Autodesk Fusion 360 part; units mm, degrees
note: some values were not read from the file. Chosen so that the rebuilt part matches the saved one: which face or edge a step refers to; which pieces of a blend or face edit are solid.
(part 2 of 2)
extrude "Extrusion30" add sketch "Skizze30" along normal blind 1 contours L54 L59 L60 L61 L62 L63 bodies 1
sketch "Skizze31" plane through (0, 1, 0) normal (0, 1, 0) x (-1, 0, 0)
  line L0 (-3.5, 38.5) -> (-3.5, 36.5)
  line L1 (-3.5, 36.5) -> (-5.5, 36.5)
  line L2 (-5.5, 36.5) -> (-5.5, 34)
  line L3 (-5.5, 34) -> (-6, 34)
  line L4 (-6, 34) -> (-6, 39)
  line L5 (-6, 39) -> (-1, 39)
  line L6 (-1, 39) -> (-1, 38.5)
  line L7 (-1, 38.5) -> (-3.5, 38.5)
  line L8 (10.5, 34) -> (10.5, 38.5)
  line L9 (10.5, 38.5) -> (6, 38.5)
  line L10 (6, 38.5) -> (6, 39)
  line L11 (6, 39) -> (11, 39)
  line L12 (11, 39) -> (11, 34)
  line L13 (11, 34) -> (10.5, 34)
  line L14 (-5.5, 8.9372) -> (-5.5, 4.5)
  line L15 (-5.5, 4.5) -> (-1, 4.5)
  line L16 (-1, 4.5) -> (-1, 4)
  line L17 (-1, 4) -> (-6, 4)
  line L18 (-6, 4) -> (-6, 8.9372)
  line L19 (-6, 8.9372) -> (-5.5, 8.9372)
  line L20 (-132.5, 5.5) -> (-132.5, 3.5)
  line L21 (-132.5, 3.5) -> (-130, 3.5)
  line L22 (-130, 3.5) -> (-130, 3)
  line L23 (-130, 3) -> (-135, 3)
  line L24 (-135, 3) -> (-135, 0)
  line L25 (-135, 0) -> (17, 0)
  line L26 (17, 0) -> (17, 40)
  line L27 (17, 40) -> (0, 40)
  line L28 (0, 40) -> (0, 68.5)
  line L29 (0, 68.5) -> (-114.094, 68.5)
  line L30 (-114.094, 68.5) -> (-114.094, 63.5)
  line L31 (-114.094, 63.5) -> (-114.594, 63.5)
  line L32 (-114.594, 63.5) -> (-114.594, 66)
  line L33 (-114.594, 66) -> (-116.594, 66)
  line L34 (-116.594, 66) -> (-116.594, 68)
  line L35 (-116.594, 68) -> (-119.094, 68)
  line L36 (-119.094, 68) -> (-119.094, 68.5)
  line L37 (-119.094, 68.5) -> (-130, 68.5)
  line L38 (-130, 68.5) -> (-130, 68)
  line L39 (-130, 68) -> (-132.5, 68)
  line L40 (-132.5, 68) -> (-132.5, 66)
  line L41 (-132.5, 66) -> (-134.5, 66)
  line L42 (-134.5, 66) -> (-134.5, 63.5)
  line L43 (-134.5, 63.5) -> (-135, 63.5)
  line L44 (-135, 63.5) -> (-135, 8.5)
  line L45 (-135, 8.5) -> (-134.5, 8.5)
  line L46 (-134.5, 8.5) -> (-134.5, 5.5)
  line L47 (-134.5, 5.5) -> (-132.5, 5.5)
  line L48 (-116.5, 3.5) -> (-116.5, 5.5)
  line L49 (-116.5, 5.5) -> (-114.5, 5.5)
  line L50 (-114.5, 5.5) -> (-114.5, 8)
  line L51 (-114.5, 8) -> (-114, 8)
  line L52 (-114, 8) -> (-114, 3)
  line L53 (-114, 3) -> (-119, 3)
  line L54 (-119, 3) -> (-119, 3.5)
  line L55 (-119, 3.5) -> (-116.5, 3.5)
  circle A0 centre (-9.9603, 7.5483) radius 1.25
  circle A1 centre (-111.4603, 7.5483) radius 1.25
  circle A2 centre (-9.9603, 64.0483) radius 1.25
  circle A3 centre (-111.4603, 64.0483) radius 1.25
  line L56 (10.5, 4.5) -> (10.5, 9)
  line L57 (10.5, 9) -> (11, 9)
  line L58 (11, 9) -> (11, 4)
  line L59 (11, 4) -> (6, 4)
  line L60 (6, 4) -> (6, 4.5)
  line L61 (6, 4.5) -> (10.5, 4.5)
  line L62 (10.5, 38.5) -> (8.5, 38.5)
  line L63 (8.5, 38.5) -> (8.5, 36.5)
  line L64 (8.5, 36.5) -> (10.5, 36.5)
  line L65 (10.5, 36.5) -> (10.5, 38.5)
  dimension "d132" = 2
  dimension "d133" = 2
  constraint horizontal L62
  constraint vertical L63
  constraint horizontal L64
  constraint vertical L65
  constraint coincident L8.end L9.start
  measures "d132" distance of L8.end L62.end
  measures "d133" distance of L8.end L64.end
extrude "Extrusion31" add sketch "Skizze31" along normal blind 1 contours L8 L9 L62 L63 L64 L65 bodies 1
sketch "Skizze32" plane through (0, 1, 0) normal (0, 1, 0) x (-1, 0, 0)
  line L0 (8.5, 36.5) -> (8.5, 38.5)
  line L1 (8.5, 38.5) -> (6, 38.5)
  line L2 (6, 38.5) -> (6, 39)
  line L3 (6, 39) -> (11, 39)
  line L4 (11, 39) -> (11, 34)
  line L5 (11, 34) -> (10.5, 34)
  line L6 (10.5, 34) -> (10.5, 36.5)
  line L7 (10.5, 36.5) -> (8.5, 36.5)
  line L8 (-3.5, 38.5) -> (-3.5, 36.5)
  line L9 (-3.5, 36.5) -> (-5.5, 36.5)
  line L10 (-5.5, 36.5) -> (-5.5, 34)
  line L11 (-5.5, 34) -> (-6, 34)
  line L12 (-6, 34) -> (-6, 39)
  line L13 (-6, 39) -> (-1, 39)
  line L14 (-1, 39) -> (-1, 38.5)
  line L15 (-1, 38.5) -> (-3.5, 38.5)
  line L16 (-5.5, 8.9372) -> (-5.5, 4.5)
  line L17 (-5.5, 4.5) -> (-1, 4.5)
  line L18 (-1, 4.5) -> (-1, 4)
  line L19 (-1, 4) -> (-6, 4)
  line L20 (-6, 4) -> (-6, 8.9372)
  line L21 (-6, 8.9372) -> (-5.5, 8.9372)
  line L22 (-132.5, 5.5) -> (-132.5, 3.5)
  line L23 (-132.5, 3.5) -> (-130, 3.5)
  line L24 (-130, 3.5) -> (-130, 3)
  line L25 (-130, 3) -> (-135, 3)
  line L26 (-135, 3) -> (-135, 0)
  line L27 (-135, 0) -> (17, 0)
  line L28 (17, 0) -> (17, 40)
  line L29 (17, 40) -> (0, 40)
  line L30 (0, 40) -> (0, 68.5)
  line L31 (0, 68.5) -> (-114.094, 68.5)
  line L32 (-114.094, 68.5) -> (-114.094, 63.5)
  line L33 (-114.094, 63.5) -> (-114.594, 63.5)
  line L34 (-114.594, 63.5) -> (-114.594, 66)
  line L35 (-114.594, 66) -> (-116.594, 66)
  line L36 (-116.594, 66) -> (-116.594, 68)
  line L37 (-116.594, 68) -> (-119.094, 68)
  line L38 (-119.094, 68) -> (-119.094, 68.5)
  line L39 (-119.094, 68.5) -> (-130, 68.5)
  line L40 (-130, 68.5) -> (-130, 68)
  line L41 (-130, 68) -> (-132.5, 68)
  line L42 (-132.5, 68) -> (-132.5, 66)
  line L43 (-132.5, 66) -> (-134.5, 66)
  line L44 (-134.5, 66) -> (-134.5, 63.5)
  line L45 (-134.5, 63.5) -> (-135, 63.5)
  line L46 (-135, 63.5) -> (-135, 8.5)
  line L47 (-135, 8.5) -> (-134.5, 8.5)
  line L48 (-134.5, 8.5) -> (-134.5, 5.5)
  line L49 (-134.5, 5.5) -> (-132.5, 5.5)
  line L50 (-116.5, 3.5) -> (-116.5, 5.5)
  line L51 (-116.5, 5.5) -> (-114.5, 5.5)
  line L52 (-114.5, 5.5) -> (-114.5, 8)
  line L53 (-114.5, 8) -> (-114, 8)
  line L54 (-114, 8) -> (-114, 3)
  line L55 (-114, 3) -> (-119, 3)
  line L56 (-119, 3) -> (-119, 3.5)
  line L57 (-119, 3.5) -> (-116.5, 3.5)
  circle A0 centre (-9.9603, 7.5483) radius 1.25
  circle A1 centre (-111.4603, 7.5483) radius 1.25
  circle A2 centre (-9.9603, 64.0483) radius 1.25
  circle A3 centre (-111.4603, 64.0483) radius 1.25
  line L58 (10.5, 4.5) -> (10.5, 9)
  line L59 (10.5, 9) -> (11, 9)
  line L60 (11, 9) -> (11, 4)
  line L61 (11, 4) -> (6, 4)
  line L62 (6, 4) -> (6, 4.5)
  line L63 (6, 4.5) -> (10.5, 4.5)
  line L64 (10.5, 4.5) -> (8.5, 4.5)
  line L65 (8.5, 4.5) -> (8.5, 6.5)
  line L66 (8.5, 6.5) -> (10.5, 6.5)
  line L67 (10.5, 6.5) -> (10.5, 4.5)
  dimension "d136" = 2
  dimension "d137" = 2
  constraint horizontal L64
  constraint vertical L65
  constraint horizontal L66
  constraint vertical L67
  constraint coincident L58.start L63.end
  measures "d136" distance of L58.start L64.end
  measures "d137" distance of L58.start L66.end
extrude "Extrusion32" add sketch "Skizze32" along normal blind 1 contours L58 L63 L64 L65 L66 L67 bodies 1
sketch "Skizze33" plane through (0, 1, 0) normal (0, 1, 0) x (-1, 0, 0)
  line L0 (8.5, 4.5) -> (8.5, 6.5)
  line L1 (8.5, 6.5) -> (10.5, 6.5)
  line L2 (10.5, 6.5) -> (10.5, 9)
  line L3 (10.5, 9) -> (11, 9)
  line L4 (11, 9) -> (11, 4)
  line L5 (11, 4) -> (6, 4)
  line L6 (6, 4) -> (6, 4.5)
  line L7 (6, 4.5) -> (8.5, 4.5)
  circle A0 centre (-111.4603, 64.0483) radius 1.25
  circle A1 centre (-9.9603, 64.0483) radius 1.25
  circle A2 centre (-111.4603, 7.5483) radius 1.25
  circle A3 centre (-9.9603, 7.5483) radius 1.25
  line L8 (-116.5, 3.5) -> (-116.5, 5.5)
  line L9 (-116.5, 5.5) -> (-114.5, 5.5)
  line L10 (-114.5, 5.5) -> (-114.5, 8)
  line L11 (-114.5, 8) -> (-114, 8)
  line L12 (-114, 8) -> (-114, 3)
  line L13 (-114, 3) -> (-119, 3)
  line L14 (-119, 3) -> (-119, 3.5)
  line L15 (-119, 3.5) -> (-116.5, 3.5)
  line L16 (-132.5, 5.5) -> (-132.5, 3.5)
  line L17 (-132.5, 3.5) -> (-130, 3.5)
  line L18 (-130, 3.5) -> (-130, 3)
  line L19 (-130, 3) -> (-135, 3)
  line L20 (-135, 3) -> (-135, 0)
  line L21 (-135, 0) -> (17, 0)
  line L22 (17, 0) -> (17, 40)
  line L23 (17, 40) -> (0, 40)
  line L24 (0, 40) -> (0, 68.5)
  line L25 (0, 68.5) -> (-114.094, 68.5)
  line L26 (-114.094, 68.5) -> (-114.094, 63.5)
  line L27 (-114.094, 63.5) -> (-114.594, 63.5)
  line L28 (-114.594, 63.5) -> (-114.594, 66)
  line L29 (-114.594, 66) -> (-116.594, 66)
  line L30 (-116.594, 66) -> (-116.594, 68)
  line L31 (-116.594, 68) -> (-119.094, 68)
  line L32 (-119.094, 68) -> (-119.094, 68.5)
  line L33 (-119.094, 68.5) -> (-130, 68.5)
  line L34 (-130, 68.5) -> (-130, 68)
  line L35 (-130, 68) -> (-132.5, 68)
  line L36 (-132.5, 68) -> (-132.5, 66)
  line L37 (-132.5, 66) -> (-134.5, 66)
  line L38 (-134.5, 66) -> (-134.5, 63.5)
  line L39 (-134.5, 63.5) -> (-135, 63.5)
  line L40 (-135, 63.5) -> (-135, 8.5)
  line L41 (-135, 8.5) -> (-134.5, 8.5)
  line L42 (-134.5, 8.5) -> (-134.5, 5.5)
  line L43 (-134.5, 5.5) -> (-132.5, 5.5)
  line L44 (-5.5, 8.9372) -> (-5.5, 4.5)
  line L45 (-5.5, 4.5) -> (-1, 4.5)
  line L46 (-1, 4.5) -> (-1, 4)
  line L47 (-1, 4) -> (-6, 4)
  line L48 (-6, 4) -> (-6, 8.9372)
  line L49 (-6, 8.9372) -> (-5.5, 8.9372)
  line L50 (-3.5, 38.5) -> (-3.5, 36.5)
  line L51 (-3.5, 36.5) -> (-5.5, 36.5)
  line L52 (-5.5, 36.5) -> (-5.5, 34)
  line L53 (-5.5, 34) -> (-6, 34)
  line L54 (-6, 34) -> (-6, 39)
  line L55 (-6, 39) -> (-1, 39)
  line L56 (-1, 39) -> (-1, 38.5)
  line L57 (-1, 38.5) -> (-3.5, 38.5)
  line L58 (8.5, 36.5) -> (8.5, 38.5)
  line L59 (8.5, 38.5) -> (6, 38.5)
  line L60 (6, 38.5) -> (6, 39)
  line L61 (6, 39) -> (11, 39)
  line L62 (11, 39) -> (11, 34)
  line L63 (11, 34) -> (10.5, 34)
  line L64 (10.5, 34) -> (10.5, 36.5)
  line L65 (10.5, 36.5) -> (8.5, 36.5)
  line L66 (-5.5, 4.5) -> (-3.5, 4.5)
  line L67 (-3.5, 4.5) -> (-3.5, 6.5)
  line L68 (-3.5, 6.5) -> (-5.5, 6.5)
  line L69 (-5.5, 6.5) -> (-5.5, 4.5)
  dimension "d140" = 2
  dimension "d141" = 2
  constraint horizontal L66
  constraint vertical L67
  constraint horizontal L68
  constraint vertical L69
  constraint coincident L44.end L45.start
  measures "d140" distance of L44.end L66.end
  measures "d141" distance of L44.end L68.end
extrude "Extrusion33" add sketch "Skizze33" along normal blind 1 contours L44 L45 L66 L67 L68 L69 bodies 1
sketch "Skizze34" plane through (0, 1, 0) normal (0, 1, 0) x (-1, 0, 0)
  line L0 (-3.5, 6.5) -> (-3.5, 4.5)
  line L1 (-3.5, 4.5) -> (-1, 4.5)
  line L2 (-1, 4.5) -> (-1, 4)
  line L3 (-1, 4) -> (-6, 4)
  line L4 (-6, 4) -> (-6, 8.9372)
  line L5 (-6, 8.9372) -> (-5.5, 8.9372)
  line L6 (-5.5, 8.9372) -> (-5.5, 6.5)
  line L7 (-5.5, 6.5) -> (-3.5, 6.5)
  line L8 (8.5, 4.5) -> (8.5, 6.5)
  line L9 (8.5, 6.5) -> (10.5, 6.5)
  line L10 (10.5, 6.5) -> (10.5, 9)
  line L11 (10.5, 9) -> (11, 9)
  line L12 (11, 9) -> (11, 4)
  line L13 (11, 4) -> (6, 4)
  line L14 (6, 4) -> (6, 4.5)
  line L15 (6, 4.5) -> (8.5, 4.5)
  circle A0 centre (-111.4603, 64.0483) radius 1.25
  circle A1 centre (-9.9603, 64.0483) radius 1.25
  circle A2 centre (-111.4603, 7.5483) radius 1.25
  circle A3 centre (-9.9603, 7.5483) radius 1.25
  line L16 (-116.5, 3.5) -> (-116.5, 5.5)
  line L17 (-116.5, 5.5) -> (-114.5, 5.5)
  line L18 (-114.5, 5.5) -> (-114.5, 8)
  line L19 (-114.5, 8) -> (-114, 8)
  line L20 (-114, 8) -> (-114, 3)
  line L21 (-114, 3) -> (-119, 3)
  line L22 (-119, 3) -> (-119, 3.5)
  line L23 (-119, 3.5) -> (-116.5, 3.5)
  line L24 (-132.5, 5.5) -> (-132.5, 3.5)
  line L25 (-132.5, 3.5) -> (-130, 3.5)
  line L26 (-130, 3.5) -> (-130, 3)
  line L27 (-130, 3) -> (-135, 3)
  line L28 (-135, 3) -> (-135, 0)
  line L29 (-135, 0) -> (17, 0)
  line L30 (17, 0) -> (17, 40)
  line L31 (17, 40) -> (0, 40)
  line L32 (0, 40) -> (0, 68.5)
  line L33 (0, 68.5) -> (-114.094, 68.5)
  line L34 (-114.094, 68.5) -> (-114.094, 63.5)
  line L35 (-114.094, 63.5) -> (-114.594, 63.5)
  line L36 (-114.594, 63.5) -> (-114.594, 66)
  line L37 (-114.594, 66) -> (-116.594, 66)
  line L38 (-116.594, 66) -> (-116.594, 68)
  line L39 (-116.594, 68) -> (-119.094, 68)
  line L40 (-119.094, 68) -> (-119.094, 68.5)
  line L41 (-119.094, 68.5) -> (-130, 68.5)
  line L42 (-130, 68.5) -> (-130, 68)
  line L43 (-130, 68) -> (-132.5, 68)
  line L44 (-132.5, 68) -> (-132.5, 66)
  line L45 (-132.5, 66) -> (-134.5, 66)
  line L46 (-134.5, 66) -> (-134.5, 63.5)
  line L47 (-134.5, 63.5) -> (-135, 63.5)
  line L48 (-135, 63.5) -> (-135, 8.5)
  line L49 (-135, 8.5) -> (-134.5, 8.5)
  line L50 (-134.5, 8.5) -> (-134.5, 5.5)
  line L51 (-134.5, 5.5) -> (-132.5, 5.5)
  line L52 (-3.5, 38.5) -> (-3.5, 36.5)
  line L53 (-3.5, 36.5) -> (-5.5, 36.5)
  line L54 (-5.5, 36.5) -> (-5.5, 34)
  line L55 (-5.5, 34) -> (-6, 34)
  line L56 (-6, 34) -> (-6, 39)
  line L57 (-6, 39) -> (-1, 39)
  line L58 (-1, 39) -> (-1, 38.5)
  line L59 (-1, 38.5) -> (-3.5, 38.5)
  line L60 (8.5, 36.5) -> (8.5, 38.5)
  line L61 (8.5, 38.5) -> (6, 38.5)
  line L62 (6, 38.5) -> (6, 39)
  line L63 (6, 39) -> (11, 39)
  line L64 (11, 39) -> (11, 34)
  line L65 (11, 34) -> (10.5, 34)
  line L66 (10.5, 34) -> (10.5, 36.5)
  line L67 (10.5, 36.5) -> (8.5, 36.5)
  line L68 (16.5, 0.5) -> (-134.5, 0.5)
  line L69 (-134.5, 0.5) -> (-134.5, 1)
  line L70 (-134.5, 1) -> (16.5, 1)
  line L71 (16.5, 1) -> (16.5, 0.5)
  dimension "d144" = 151
  dimension "d145" = 0.5
  constraint horizontal L68
  constraint vertical L69
  constraint horizontal L70
  constraint vertical L71
  measures "d144" distance of L68.start L68.end
  measures "d145" distance of L68.start L70.end
extrude "Extrusion34" add sketch "Skizze34" along normal blind 10 contours L68 L69 L70 L71 bodies 1
sketch "Skizze35" plane through (0, 1, 0) normal (0, 1, 0) x (-1, 0, 0)
  line L0 (16.5, 1) -> (16.5, 0.5)
  line L1 (16.5, 0.5) -> (-134.5, 0.5)
  line L2 (-134.5, 0.5) -> (-134.5, 1)
  line L3 (-134.5, 1) -> (16.5, 1)
  line L4 (-3.5, 6.5) -> (-3.5, 4.5)
  line L5 (-3.5, 4.5) -> (-1, 4.5)
  line L6 (-1, 4.5) -> (-1, 4)
  line L7 (-1, 4) -> (-6, 4)
  line L8 (-6, 4) -> (-6, 8.9372)
  line L9 (-6, 8.9372) -> (-5.5, 8.9372)
  line L10 (-5.5, 8.9372) -> (-5.5, 6.5)
  line L11 (-5.5, 6.5) -> (-3.5, 6.5)
  line L12 (8.5, 4.5) -> (8.5, 6.5)
  line L13 (8.5, 6.5) -> (10.5, 6.5)
  line L14 (10.5, 6.5) -> (10.5, 9)
  line L15 (10.5, 9) -> (11, 9)
  line L16 (11, 9) -> (11, 4)
  line L17 (11, 4) -> (6, 4)
  line L18 (6, 4) -> (6, 4.5)
  line L19 (6, 4.5) -> (8.5, 4.5)
  circle A0 centre (-111.4603, 64.0483) radius 1.25
  circle A1 centre (-9.9603, 64.0483) radius 1.25
  circle A2 centre (-111.4603, 7.5483) radius 1.25
  circle A3 centre (-9.9603, 7.5483) radius 1.25
  line L20 (-116.5, 3.5) -> (-116.5, 5.5)
  line L21 (-116.5, 5.5) -> (-114.5, 5.5)
  line L22 (-114.5, 5.5) -> (-114.5, 8)
  line L23 (-114.5, 8) -> (-114, 8)
  line L24 (-114, 8) -> (-114, 3)
  line L25 (-114, 3) -> (-119, 3)
  line L26 (-119, 3) -> (-119, 3.5)
  line L27 (-119, 3.5) -> (-116.5, 3.5)
  line L28 (-132.5, 5.5) -> (-132.5, 3.5)
  line L29 (-132.5, 3.5) -> (-130, 3.5)
  line L30 (-130, 3.5) -> (-130, 3)
  line L31 (-130, 3) -> (-135, 3)
  line L32 (-135, 3) -> (-135, 0)
  line L33 (-135, 0) -> (17, 0)
  line L34 (17, 0) -> (17, 40)
  line L35 (17, 40) -> (0, 40)
  line L36 (0, 40) -> (0, 68.5)
  line L37 (0, 68.5) -> (-114.094, 68.5)
  line L38 (-114.094, 68.5) -> (-114.094, 63.5)
  line L39 (-114.094, 63.5) -> (-114.594, 63.5)
  line L40 (-114.594, 63.5) -> (-114.594, 66)
  line L41 (-114.594, 66) -> (-116.594, 66)
  line L42 (-116.594, 66) -> (-116.594, 68)
  line L43 (-116.594, 68) -> (-119.094, 68)
  line L44 (-119.094, 68) -> (-119.094, 68.5)
  line L45 (-119.094, 68.5) -> (-130, 68.5)
  line L46 (-130, 68.5) -> (-130, 68)
  line L47 (-130, 68) -> (-132.5, 68)
  line L48 (-132.5, 68) -> (-132.5, 66)
  line L49 (-132.5, 66) -> (-134.5, 66)
  line L50 (-134.5, 66) -> (-134.5, 63.5)
  line L51 (-134.5, 63.5) -> (-135, 63.5)
  line L52 (-135, 63.5) -> (-135, 8.5)
  line L53 (-135, 8.5) -> (-134.5, 8.5)
  line L54 (-134.5, 8.5) -> (-134.5, 5.5)
  line L55 (-134.5, 5.5) -> (-132.5, 5.5)
  line L56 (-3.5, 38.5) -> (-3.5, 36.5)
  line L57 (-3.5, 36.5) -> (-5.5, 36.5)
  line L58 (-5.5, 36.5) -> (-5.5, 34)
  line L59 (-5.5, 34) -> (-6, 34)
  line L60 (-6, 34) -> (-6, 39)
  line L61 (-6, 39) -> (-1, 39)
  line L62 (-1, 39) -> (-1, 38.5)
  line L63 (-1, 38.5) -> (-3.5, 38.5)
  line L64 (8.5, 36.5) -> (8.5, 38.5)
  line L65 (8.5, 38.5) -> (6, 38.5)
  line L66 (6, 38.5) -> (6, 39)
  line L67 (6, 39) -> (11, 39)
  line L68 (11, 39) -> (11, 34)
  line L69 (11, 34) -> (10.5, 34)
  line L70 (10.5, 34) -> (10.5, 36.5)
  line L71 (10.5, 36.5) -> (8.5, 36.5)
  line L72 (-134.5, 1) -> (-134, 1)
  line L73 (-134, 1) -> (-134, 3)
  line L74 (-134, 3) -> (-134.5, 3)
  line L75 (-134.5, 3) -> (-134.5, 1)
  constraint horizontal L72
  constraint vertical L73
  constraint horizontal L74
  constraint vertical L75
  constraint coincident L31 L73.end
  constraint coincident L2.end L3.start
extrude "Extrusion35" add sketch "Skizze35" along normal blind 10 contours L3 L31 L72 L73 L74 L75 bodies 1
sketch "Skizze36" plane through (0, 1, 0) normal (0, 1, 0) x (-1, 0, 0)
  line L0 (8.5, 36.5) -> (8.5, 38.5)
  line L1 (8.5, 38.5) -> (6, 38.5)
  line L2 (6, 38.5) -> (6, 39)
  line L3 (6, 39) -> (11, 39)
  line L4 (11, 39) -> (11, 34)
  line L5 (11, 34) -> (10.5, 34)
  line L6 (10.5, 34) -> (10.5, 36.5)
  line L7 (10.5, 36.5) -> (8.5, 36.5)
  line L8 (-3.5, 38.5) -> (-3.5, 36.5)
  line L9 (-3.5, 36.5) -> (-5.5, 36.5)
  line L10 (-5.5, 36.5) -> (-5.5, 34)
  line L11 (-5.5, 34) -> (-6, 34)
  line L12 (-6, 34) -> (-6, 39)
  line L13 (-6, 39) -> (-1, 39)
  line L14 (-1, 39) -> (-1, 38.5)
  line L15 (-1, 38.5) -> (-3.5, 38.5)
  line L16 (-116.5, 3.5) -> (-116.5, 5.5)
  line L17 (-116.5, 5.5) -> (-114.5, 5.5)
  line L18 (-114.5, 5.5) -> (-114.5, 8)
  line L19 (-114.5, 8) -> (-114, 8)
  line L20 (-114, 8) -> (-114, 3)
  line L21 (-114, 3) -> (-119, 3)
  line L22 (-119, 3) -> (-119, 3.5)
  line L23 (-119, 3.5) -> (-116.5, 3.5)
  circle A0 centre (-9.9603, 7.5483) radius 1.25
  circle A1 centre (-111.4603, 7.5483) radius 1.25
  circle A2 centre (-9.9603, 64.0483) radius 1.25
  circle A3 centre (-111.4603, 64.0483) radius 1.25
  line L24 (8.5, 4.5) -> (8.5, 6.5)
  line L25 (8.5, 6.5) -> (10.5, 6.5)
  line L26 (10.5, 6.5) -> (10.5, 9)
  line L27 (10.5, 9) -> (11, 9)
  line L28 (11, 9) -> (11, 4)
  line L29 (11, 4) -> (6, 4)
  line L30 (6, 4) -> (6, 4.5)
  line L31 (6, 4.5) -> (8.5, 4.5)
  line L32 (-3.5, 6.5) -> (-3.5, 4.5)
  line L33 (-3.5, 4.5) -> (-1, 4.5)
  line L34 (-1, 4.5) -> (-1, 4)
  line L35 (-1, 4) -> (-6, 4)
  line L36 (-6, 4) -> (-6, 8.9372)
  line L37 (-6, 8.9372) -> (-5.5, 8.9372)
  line L38 (-5.5, 8.9372) -> (-5.5, 6.5)
  line L39 (-5.5, 6.5) -> (-3.5, 6.5)
  line L40 (-134, 3) -> (-134, 1)
  line L41 (-134, 1) -> (16.5, 1)
  line L42 (16.5, 1) -> (16.5, 0.5)
  line L43 (16.5, 0.5) -> (-134.5, 0.5)
  line L44 (-134.5, 0.5) -> (-134.5, 3)
  line L45 (-134.5, 3) -> (-135, 3)
  line L46 (-135, 3) -> (-135, 0)
  line L47 (-135, 0) -> (17, 0)
  line L48 (17, 0) -> (17, 40)
  line L49 (17, 40) -> (0, 40)
  line L50 (0, 40) -> (0, 68.5)
  line L51 (0, 68.5) -> (-114.094, 68.5)
  line L52 (-114.094, 68.5) -> (-114.094, 63.5)
  line L53 (-114.094, 63.5) -> (-114.594, 63.5)
  line L54 (-114.594, 63.5) -> (-114.594, 66)
  line L55 (-114.594, 66) -> (-116.594, 66)
  line L56 (-116.594, 66) -> (-116.594, 68)
  line L57 (-116.594, 68) -> (-119.094, 68)
  line L58 (-119.094, 68) -> (-119.094, 68.5)
  line L59 (-119.094, 68.5) -> (-130, 68.5)
  line L60 (-130, 68.5) -> (-130, 68)
  line L61 (-130, 68) -> (-132.5, 68)
  line L62 (-132.5, 68) -> (-132.5, 66)
  line L63 (-132.5, 66) -> (-134.5, 66)
  line L64 (-134.5, 66) -> (-134.5, 63.5)
  line L65 (-134.5, 63.5) -> (-135, 63.5)
  line L66 (-135, 63.5) -> (-135, 8.5)
  line L67 (-135, 8.5) -> (-134.5, 8.5)
  line L68 (-134.5, 8.5) -> (-134.5, 5.5)
  line L69 (-134.5, 5.5) -> (-132.5, 5.5)
  line L70 (-132.5, 5.5) -> (-132.5, 3.5)
  line L71 (-132.5, 3.5) -> (-130, 3.5)
  line L72 (-130, 3.5) -> (-130, 3)
  line L73 (-130, 3) -> (-134, 3)
  line L74 (16.5, 39.5) -> (16, 39.5)
  line L75 (16, 39.5) -> (16, 1)
  line L76 (16, 1) -> (16.5, 1)
  line L77 (16.5, 1) -> (16.5, 39.5)
  dimension "d150" = 0.5
  constraint horizontal L74
  constraint vertical L75
  constraint horizontal L76
  constraint vertical L77
  measures "d150" distance of L74.start L74.end
extrude "Extrusion36" add sketch "Skizze36" along normal blind 10 contours L41 L74 L75 L76 L77 bodies 1
sketch "Skizze37" plane through (0, 1, 0) normal (0, 1, 0) x (-1, 0, 0)
  line L0 (16, 1) -> (16, 39.5)
  line L1 (16, 39.5) -> (16.5, 39.5)
  line L2 (16.5, 39.5) -> (16.5, 0.5)
  line L3 (16.5, 0.5) -> (-134.5, 0.5)
  line L4 (-134.5, 0.5) -> (-134.5, 3)
  line L5 (-134.5, 3) -> (-135, 3)
  line L6 (-135, 3) -> (-135, 0)
  line L7 (-135, 0) -> (17, 0)
  line L8 (17, 0) -> (17, 40)
  line L9 (17, 40) -> (0, 40)
  line L10 (0, 40) -> (0, 68.5)
  line L11 (0, 68.5) -> (-114.094, 68.5)
  line L12 (-114.094, 68.5) -> (-114.094, 63.5)
  line L13 (-114.094, 63.5) -> (-114.594, 63.5)
  line L14 (-114.594, 63.5) -> (-114.594, 66)
  line L15 (-114.594, 66) -> (-116.594, 66)
  line L16 (-116.594, 66) -> (-116.594, 68)
  line L17 (-116.594, 68) -> (-119.094, 68)
  line L18 (-119.094, 68) -> (-119.094, 68.5)
  line L19 (-119.094, 68.5) -> (-130, 68.5)
  line L20 (-130, 68.5) -> (-130, 68)
  line L21 (-130, 68) -> (-132.5, 68)
  line L22 (-132.5, 68) -> (-132.5, 66)
  line L23 (-132.5, 66) -> (-134.5, 66)
  line L24 (-134.5, 66) -> (-134.5, 63.5)
  line L25 (-134.5, 63.5) -> (-135, 63.5)
  line L26 (-135, 63.5) -> (-135, 8.5)
  line L27 (-135, 8.5) -> (-134.5, 8.5)
  line L28 (-134.5, 8.5) -> (-134.5, 5.5)
  line L29 (-134.5, 5.5) -> (-132.5, 5.5)
  line L30 (-132.5, 5.5) -> (-132.5, 3.5)
  line L31 (-132.5, 3.5) -> (-130, 3.5)
  line L32 (-130, 3.5) -> (-130, 3)
  line L33 (-130, 3) -> (-134, 3)
  line L34 (-134, 3) -> (-134, 1)
  line L35 (-134, 1) -> (16, 1)
  line L36 (-3.5, 6.5) -> (-3.5, 4.5)
  line L37 (-3.5, 4.5) -> (-1, 4.5)
  line L38 (-1, 4.5) -> (-1, 4)
  line L39 (-1, 4) -> (-6, 4)
  line L40 (-6, 4) -> (-6, 8.9372)
  line L41 (-6, 8.9372) -> (-5.5, 8.9372)
  line L42 (-5.5, 8.9372) -> (-5.5, 6.5)
  line L43 (-5.5, 6.5) -> (-3.5, 6.5)
  line L44 (8.5, 4.5) -> (8.5, 6.5)
  line L45 (8.5, 6.5) -> (10.5, 6.5)
  line L46 (10.5, 6.5) -> (10.5, 9)
  line L47 (10.5, 9) -> (11, 9)
  line L48 (11, 9) -> (11, 4)
  line L49 (11, 4) -> (6, 4)
  line L50 (6, 4) -> (6, 4.5)
  line L51 (6, 4.5) -> (8.5, 4.5)
  circle A0 centre (-111.4603, 64.0483) radius 1.25
  circle A1 centre (-9.9603, 64.0483) radius 1.25
  circle A2 centre (-111.4603, 7.5483) radius 1.25
  circle A3 centre (-9.9603, 7.5483) radius 1.25
  line L52 (-116.5, 3.5) -> (-116.5, 5.5)
  line L53 (-116.5, 5.5) -> (-114.5, 5.5)
  line L54 (-114.5, 5.5) -> (-114.5, 8)
  line L55 (-114.5, 8) -> (-114, 8)
  line L56 (-114, 8) -> (-114, 3)
  line L57 (-114, 3) -> (-119, 3)
  line L58 (-119, 3) -> (-119, 3.5)
  line L59 (-119, 3.5) -> (-116.5, 3.5)
  line L60 (-3.5, 38.5) -> (-3.5, 36.5)
  line L61 (-3.5, 36.5) -> (-5.5, 36.5)
  line L62 (-5.5, 36.5) -> (-5.5, 34)
  line L63 (-5.5, 34) -> (-6, 34)
  line L64 (-6, 34) -> (-6, 39)
  line L65 (-6, 39) -> (-1, 39)
  line L66 (-1, 39) -> (-1, 38.5)
  line L67 (-1, 38.5) -> (-3.5, 38.5)
  line L68 (8.5, 36.5) -> (8.5, 38.5)
  line L69 (8.5, 38.5) -> (6, 38.5)
  line L70 (6, 38.5) -> (6, 39)
  line L71 (6, 39) -> (11, 39)
  line L72 (11, 39) -> (11, 34)
  line L73 (11, 34) -> (10.5, 34)
  line L74 (10.5, 34) -> (10.5, 36.5)
  line L75 (10.5, 36.5) -> (8.5, 36.5)
  line L76 (16, 39.5) -> (0, 39.5)
  line L77 (0, 39.5) -> (0, 39)
  line L78 (0, 39) -> (16, 39)
  line L79 (16, 39) -> (16, 39.5)
  constraint horizontal L76
  constraint vertical L77
  constraint horizontal L78
  constraint vertical L79
  constraint coincident L0.end L1.start
extrude "Extrusion37" add sketch "Skizze37" along normal blind 10 contours L0 L71 L76 L77 L78 L79 bodies 1
sketch "Skizze38" plane through (0, 1, 0) normal (0, 1, 0) x (-1, 0, 0)
  line L0 (-3.5, 38.5) -> (-3.5, 36.5)
  line L1 (-3.5, 36.5) -> (-5.5, 36.5)
  line L2 (-5.5, 36.5) -> (-5.5, 34)
  line L3 (-5.5, 34) -> (-6, 34)
  line L4 (-6, 34) -> (-6, 39)
  line L5 (-6, 39) -> (-1, 39)
  line L6 (-1, 39) -> (-1, 38.5)
  line L7 (-1, 38.5) -> (-3.5, 38.5)
  line L8 (-116.5, 3.5) -> (-116.5, 5.5)
  line L9 (-116.5, 5.5) -> (-114.5, 5.5)
  line L10 (-114.5, 5.5) -> (-114.5, 8)
  line L11 (-114.5, 8) -> (-114, 8)
  line L12 (-114, 8) -> (-114, 3)
  line L13 (-114, 3) -> (-119, 3)
  line L14 (-119, 3) -> (-119, 3.5)
  line L15 (-119, 3.5) -> (-116.5, 3.5)
  circle A0 centre (-9.9603, 7.5483) radius 1.25
  circle A1 centre (-111.4603, 7.5483) radius 1.25
  circle A2 centre (-9.9603, 64.0483) radius 1.25
  circle A3 centre (-111.4603, 64.0483) radius 1.25
  line L16 (8.5, 4.5) -> (8.5, 6.5)
  line L17 (8.5, 6.5) -> (10.5, 6.5)
  line L18 (10.5, 6.5) -> (10.5, 9)
  line L19 (10.5, 9) -> (11, 9)
  line L20 (11, 9) -> (11, 4)
  line L21 (11, 4) -> (6, 4)
  line L22 (6, 4) -> (6, 4.5)
  line L23 (6, 4.5) -> (8.5, 4.5)
  line L24 (-3.5, 6.5) -> (-3.5, 4.5)
  line L25 (-3.5, 4.5) -> (-1, 4.5)
  line L26 (-1, 4.5) -> (-1, 4)
  line L27 (-1, 4) -> (-6, 4)
  line L28 (-6, 4) -> (-6, 8.9372)
  line L29 (-6, 8.9372) -> (-5.5, 8.9372)
  line L30 (-5.5, 8.9372) -> (-5.5, 6.5)
  line L31 (-5.5, 6.5) -> (-3.5, 6.5)
  line L32 (6, 39) -> (0, 39)
  line L33 (0, 39) -> (0, 39.5)
  line L34 (0, 39.5) -> (16.5, 39.5)
  line L35 (16.5, 39.5) -> (16.5, 0.5)
  line L36 (16.5, 0.5) -> (-134.5, 0.5)
  line L37 (-134.5, 0.5) -> (-134.5, 3)
  line L38 (-134.5, 3) -> (-135, 3)
  line L39 (-135, 3) -> (-135, 0)
  line L40 (-135, 0) -> (17, 0)
  line L41 (17, 0) -> (17, 40)
  line L42 (17, 40) -> (0, 40)
  line L43 (0, 40) -> (0, 68.5)
  line L44 (0, 68.5) -> (-114.094, 68.5)
  line L45 (-114.094, 68.5) -> (-114.094, 63.5)
  line L46 (-114.094, 63.5) -> (-114.594, 63.5)
  line L47 (-114.594, 63.5) -> (-114.594, 66)
  line L48 (-114.594, 66) -> (-116.594, 66)
  line L49 (-116.594, 66) -> (-116.594, 68)
  line L50 (-116.594, 68) -> (-119.094, 68)
  line L51 (-119.094, 68) -> (-119.094, 68.5)
  line L52 (-119.094, 68.5) -> (-130, 68.5)
  line L53 (-130, 68.5) -> (-130, 68)
  line L54 (-130, 68) -> (-132.5, 68)
  line L55 (-132.5, 68) -> (-132.5, 66)
  line L56 (-132.5, 66) -> (-134.5, 66)
  line L57 (-134.5, 66) -> (-134.5, 63.5)
  line L58 (-134.5, 63.5) -> (-135, 63.5)
  line L59 (-135, 63.5) -> (-135, 8.5)
  line L60 (-135, 8.5) -> (-134.5, 8.5)
  line L61 (-134.5, 8.5) -> (-134.5, 5.5)
  line L62 (-134.5, 5.5) -> (-132.5, 5.5)
  line L63 (-132.5, 5.5) -> (-132.5, 3.5)
  line L64 (-132.5, 3.5) -> (-130, 3.5)
  line L65 (-130, 3.5) -> (-130, 3)
  line L66 (-130, 3) -> (-134, 3)
  line L67 (-134, 3) -> (-134, 1)
  line L68 (-134, 1) -> (16, 1)
  line L69 (16, 1) -> (16, 39)
  line L70 (16, 39) -> (11, 39)
  line L71 (11, 39) -> (11, 34)
  line L72 (11, 34) -> (10.5, 34)
  line L73 (10.5, 34) -> (10.5, 36.5)
  line L74 (10.5, 36.5) -> (8.5, 36.5)
  line L75 (8.5, 36.5) -> (8.5, 38.5)
  line L76 (8.5, 38.5) -> (6, 38.5)
  line L77 (6, 38.5) -> (6, 39)
  line L78 (-0.5, 68) -> (-1, 68)
  line L79 (-1, 68) -> (-1, 39)
  line L80 (-1, 39) -> (-0.5, 39)
  line L81 (-0.5, 39) -> (-0.5, 68)
  constraint horizontal L78
  constraint vertical L79
  constraint horizontal L80
  constraint vertical L81
  constraint coincident L5.end L6.start
extrude "Extrusion38" add sketch "Skizze38" along normal blind 10 separate body contours L78 L79 L80 L81 makes body 2
sketch "Skizze39" plane through (0, 1, 0) normal (0, 1, 0) x (-1, 0, 0)
  line L0 (-3.5, 38.5) -> (-3.5, 36.5)
  line L1 (-3.5, 36.5) -> (-5.5, 36.5)
  line L2 (-5.5, 36.5) -> (-5.5, 34)
  line L3 (-5.5, 34) -> (-6, 34)
  line L4 (-6, 34) -> (-6, 39)
  line L5 (-6, 39) -> (-1, 39)
  line L6 (-1, 39) -> (-1, 38.5)
  line L7 (-1, 38.5) -> (-3.5, 38.5)
  line L8 (-116.5, 3.5) -> (-116.5, 5.5)
  line L9 (-116.5, 5.5) -> (-114.5, 5.5)
  line L10 (-114.5, 5.5) -> (-114.5, 8)
  line L11 (-114.5, 8) -> (-114, 8)
  line L12 (-114, 8) -> (-114, 3)
  line L13 (-114, 3) -> (-119, 3)
  line L14 (-119, 3) -> (-119, 3.5)
  line L15 (-119, 3.5) -> (-116.5, 3.5)
  circle A0 centre (-9.9603, 7.5483) radius 1.25
  circle A1 centre (-111.4603, 7.5483) radius 1.25
  circle A2 centre (-9.9603, 64.0483) radius 1.25
  circle A3 centre (-111.4603, 64.0483) radius 1.25
  line L16 (8.5, 4.5) -> (8.5, 6.5)
  line L17 (8.5, 6.5) -> (10.5, 6.5)
  line L18 (10.5, 6.5) -> (10.5, 9)
  line L19 (10.5, 9) -> (11, 9)
  line L20 (11, 9) -> (11, 4)
  line L21 (11, 4) -> (6, 4)
  line L22 (6, 4) -> (6, 4.5)
  line L23 (6, 4.5) -> (8.5, 4.5)
  line L24 (-3.5, 6.5) -> (-3.5, 4.5)
  line L25 (-3.5, 4.5) -> (-1, 4.5)
  line L26 (-1, 4.5) -> (-1, 4)
  line L27 (-1, 4) -> (-6, 4)
  line L28 (-6, 4) -> (-6, 8.9372)
  line L29 (-6, 8.9372) -> (-5.5, 8.9372)
  line L30 (-5.5, 8.9372) -> (-5.5, 6.5)
  line L31 (-5.5, 6.5) -> (-3.5, 6.5)
  line L32 (6, 39) -> (0, 39)
  line L33 (0, 39) -> (0, 39.5)
  line L34 (0, 39.5) -> (16.5, 39.5)
  line L35 (16.5, 39.5) -> (16.5, 0.5)
  line L36 (16.5, 0.5) -> (-134.5, 0.5)
  line L37 (-134.5, 0.5) -> (-134.5, 3)
  line L38 (-134.5, 3) -> (-135, 3)
  line L39 (-135, 3) -> (-135, 0)
  line L40 (-135, 0) -> (17, 0)
  line L41 (17, 0) -> (17, 40)
  line L42 (17, 40) -> (0, 40)
  line L43 (0, 40) -> (0, 68.5)
  line L44 (0, 68.5) -> (-114.094, 68.5)
  line L45 (-114.094, 68.5) -> (-114.094, 63.5)
  line L46 (-114.094, 63.5) -> (-114.594, 63.5)
  line L47 (-114.594, 63.5) -> (-114.594, 66)
  line L48 (-114.594, 66) -> (-116.594, 66)
  line L49 (-116.594, 66) -> (-116.594, 68)
  line L50 (-116.594, 68) -> (-119.094, 68)
  line L51 (-119.094, 68) -> (-119.094, 68.5)
  line L52 (-119.094, 68.5) -> (-130, 68.5)
  line L53 (-130, 68.5) -> (-130, 68)
  line L54 (-130, 68) -> (-132.5, 68)
  line L55 (-132.5, 68) -> (-132.5, 66)
  line L56 (-132.5, 66) -> (-134.5, 66)
  line L57 (-134.5, 66) -> (-134.5, 63.5)
  line L58 (-134.5, 63.5) -> (-135, 63.5)
  line L59 (-135, 63.5) -> (-135, 8.5)
  line L60 (-135, 8.5) -> (-134.5, 8.5)
  line L61 (-134.5, 8.5) -> (-134.5, 5.5)
  line L62 (-134.5, 5.5) -> (-132.5, 5.5)
  line L63 (-132.5, 5.5) -> (-132.5, 3.5)
  line L64 (-132.5, 3.5) -> (-130, 3.5)
  line L65 (-130, 3.5) -> (-130, 3)
  line L66 (-130, 3) -> (-134, 3)
  line L67 (-134, 3) -> (-134, 1)
  line L68 (-134, 1) -> (16, 1)
  line L69 (16, 1) -> (16, 39)
  line L70 (16, 39) -> (11, 39)
  line L71 (11, 39) -> (11, 34)
  line L72 (11, 34) -> (10.5, 34)
  line L73 (10.5, 34) -> (10.5, 36.5)
  line L74 (10.5, 36.5) -> (8.5, 36.5)
  line L75 (8.5, 36.5) -> (8.5, 38.5)
  line L76 (8.5, 38.5) -> (6, 38.5)
  line L77 (6, 38.5) -> (6, 39)
  line L78 (-0.5, 39.5) -> (0, 39.5)
  line L79 (0, 39.5) -> (0, 39)
  line L80 (0, 39) -> (-0.5, 39)
  line L81 (-0.5, 39) -> (-0.5, 39.5)
  constraint horizontal L78
  constraint vertical L79
  constraint horizontal L80
  constraint vertical L81
  constraint coincident L32.end L33.start
extrude "Extrusion39" add sketch "Skizze39" along normal blind 10 contours L33 L78 L79 L80 L81 bodies 1 2
sketch "Skizze40" plane through (0, 1, 0) normal (0, 1, 0) x (-1, 0, 0)
  line L0 (-0.5, 68) -> (-0.5, 39.5)
  line L1 (-0.5, 39.5) -> (16.5, 39.5)
  line L2 (16.5, 39.5) -> (16.5, 0.5)
  line L3 (16.5, 0.5) -> (-134.5, 0.5)
  line L4 (-134.5, 0.5) -> (-134.5, 3)
  line L5 (-134.5, 3) -> (-135, 3)
  line L6 (-135, 3) -> (-135, 0)
  line L7 (-135, 0) -> (17, 0)
  line L8 (17, 0) -> (17, 40)
  line L9 (17, 40) -> (0, 40)
  line L10 (0, 40) -> (0, 68.5)
  line L11 (0, 68.5) -> (-114.094, 68.5)
  line L12 (-114.094, 68.5) -> (-114.094, 63.5)
  line L13 (-114.094, 63.5) -> (-114.594, 63.5)
  line L14 (-114.594, 63.5) -> (-114.594, 66)
  line L15 (-114.594, 66) -> (-116.594, 66)
  line L16 (-116.594, 66) -> (-116.594, 68)
  line L17 (-116.594, 68) -> (-119.094, 68)
  line L18 (-119.094, 68) -> (-119.094, 68.5)
  line L19 (-119.094, 68.5) -> (-130, 68.5)
  line L20 (-130, 68.5) -> (-130, 68)
  line L21 (-130, 68) -> (-132.5, 68)
  line L22 (-132.5, 68) -> (-132.5, 66)
  line L23 (-132.5, 66) -> (-134.5, 66)
  line L24 (-134.5, 66) -> (-134.5, 63.5)
  line L25 (-134.5, 63.5) -> (-135, 63.5)
  line L26 (-135, 63.5) -> (-135, 8.5)
  line L27 (-135, 8.5) -> (-134.5, 8.5)
  line L28 (-134.5, 8.5) -> (-134.5, 5.5)
  line L29 (-134.5, 5.5) -> (-132.5, 5.5)
  line L30 (-132.5, 5.5) -> (-132.5, 3.5)
  line L31 (-132.5, 3.5) -> (-130, 3.5)
  line L32 (-130, 3.5) -> (-130, 3)
  line L33 (-130, 3) -> (-134, 3)
  line L34 (-134, 3) -> (-134, 1)
  line L35 (-134, 1) -> (16, 1)
  line L36 (16, 1) -> (16, 39)
  line L37 (16, 39) -> (11, 39)
  line L38 (11, 39) -> (11, 34)
  line L39 (11, 34) -> (10.5, 34)
  line L40 (10.5, 34) -> (10.5, 36.5)
  line L41 (10.5, 36.5) -> (8.5, 36.5)
  line L42 (8.5, 36.5) -> (8.5, 38.5)
  line L43 (8.5, 38.5) -> (6, 38.5)
  line L44 (6, 38.5) -> (6, 39)
  line L45 (6, 39) -> (-1, 39)
  line L46 (-1, 39) -> (-1, 38.5)
  line L47 (-1, 38.5) -> (-3.5, 38.5)
  line L48 (-3.5, 38.5) -> (-3.5, 36.5)
  line L49 (-3.5, 36.5) -> (-5.5, 36.5)
  line L50 (-5.5, 36.5) -> (-5.5, 34)
  line L51 (-5.5, 34) -> (-6, 34)
  line L52 (-6, 34) -> (-6, 39)
  line L53 (-6, 39) -> (-1, 39)
  line L54 (-1, 39) -> (-1, 68)
  line L55 (-1, 68) -> (-0.5, 68)
  line L56 (-116.5, 3.5) -> (-116.5, 5.5)
  line L57 (-116.5, 5.5) -> (-114.5, 5.5)
  line L58 (-114.5, 5.5) -> (-114.5, 8)
  line L59 (-114.5, 8) -> (-114, 8)
  line L60 (-114, 8) -> (-114, 3)
  line L61 (-114, 3) -> (-119, 3)
  line L62 (-119, 3) -> (-119, 3.5)
  line L63 (-119, 3.5) -> (-116.5, 3.5)
  circle A0 centre (-9.9603, 7.5483) radius 1.25
  circle A1 centre (-111.4603, 7.5483) radius 1.25
  circle A2 centre (-9.9603, 64.0483) radius 1.25
  circle A3 centre (-111.4603, 64.0483) radius 1.25
  line L64 (8.5, 4.5) -> (8.5, 6.5)
  line L65 (8.5, 6.5) -> (10.5, 6.5)
  line L66 (10.5, 6.5) -> (10.5, 9)
  line L67 (10.5, 9) -> (11, 9)
  line L68 (11, 9) -> (11, 4)
  line L69 (11, 4) -> (6, 4)
  line L70 (6, 4) -> (6, 4.5)
  line L71 (6, 4.5) -> (8.5, 4.5)
  line L72 (-3.5, 6.5) -> (-3.5, 4.5)
  line L73 (-3.5, 4.5) -> (-1, 4.5)
  line L74 (-1, 4.5) -> (-1, 4)
  line L75 (-1, 4) -> (-6, 4)
  line L76 (-6, 4) -> (-6, 8.9372)
  line L77 (-6, 8.9372) -> (-5.5, 8.9372)
  line L78 (-5.5, 8.9372) -> (-5.5, 6.5)
  line L79 (-5.5, 6.5) -> (-3.5, 6.5)
  line L80 (-1, 68) -> (-114.1041, 68)
  line L81 (-114.1041, 68) -> (-114.1041, 67.5)
  line L82 (-114.1041, 67.5) -> (-1, 67.5)
  line L83 (-1, 67.5) -> (-1, 68)
  dimension "d159" = 0.5
  constraint horizontal L80
  constraint vertical L81
  constraint horizontal L82
  constraint vertical L83
  constraint coincident L54.end L55.start
  measures "d159" distance of L54.end L82.end
extrude "Extrusion40" add sketch "Skizze40" along normal blind 10 separate body contours L12 L54 L80 L82 L83 makes body 3
sketch "Skizze41" plane through (0, 1, 0) normal (0, 1, 0) x (-1, 0, 0)
  line L0 (-0.5, 68) -> (-0.5, 39.5)
  line L1 (-0.5, 39.5) -> (16.5, 39.5)
  line L2 (16.5, 39.5) -> (16.5, 0.5)
  line L3 (16.5, 0.5) -> (-134.5, 0.5)
  line L4 (-134.5, 0.5) -> (-134.5, 3)
  line L5 (-134.5, 3) -> (-135, 3)
  line L6 (-135, 3) -> (-135, 0)
  line L7 (-135, 0) -> (17, 0)
  line L8 (17, 0) -> (17, 40)
  line L9 (17, 40) -> (0, 40)
  line L10 (0, 40) -> (0, 68.5)
  line L11 (0, 68.5) -> (-114.094, 68.5)
  line L12 (-114.094, 68.5) -> (-114.094, 63.5)
  line L13 (-114.094, 63.5) -> (-114.594, 63.5)
  line L14 (-114.594, 63.5) -> (-114.594, 66)
  line L15 (-114.594, 66) -> (-116.594, 66)
  line L16 (-116.594, 66) -> (-116.594, 68)
  line L17 (-116.594, 68) -> (-119.094, 68)
  line L18 (-119.094, 68) -> (-119.094, 68.5)
  line L19 (-119.094, 68.5) -> (-130, 68.5)
  line L20 (-130, 68.5) -> (-130, 68)
  line L21 (-130, 68) -> (-132.5, 68)
  line L22 (-132.5, 68) -> (-132.5, 66)
  line L23 (-132.5, 66) -> (-134.5, 66)
  line L24 (-134.5, 66) -> (-134.5, 63.5)
  line L25 (-134.5, 63.5) -> (-135, 63.5)
  line L26 (-135, 63.5) -> (-135, 8.5)
  line L27 (-135, 8.5) -> (-134.5, 8.5)
  line L28 (-134.5, 8.5) -> (-134.5, 5.5)
  line L29 (-134.5, 5.5) -> (-132.5, 5.5)
  line L30 (-132.5, 5.5) -> (-132.5, 3.5)
  line L31 (-132.5, 3.5) -> (-130, 3.5)
  line L32 (-130, 3.5) -> (-130, 3)
  line L33 (-130, 3) -> (-134, 3)
  line L34 (-134, 3) -> (-134, 1)
  line L35 (-134, 1) -> (16, 1)
  line L36 (16, 1) -> (16, 39)
  line L37 (16, 39) -> (11, 39)
  line L38 (11, 39) -> (11, 34)
  line L39 (11, 34) -> (10.5, 34)
  line L40 (10.5, 34) -> (10.5, 36.5)
  line L41 (10.5, 36.5) -> (8.5, 36.5)
  line L42 (8.5, 36.5) -> (8.5, 38.5)
  line L43 (8.5, 38.5) -> (6, 38.5)
  line L44 (6, 38.5) -> (6, 39)
  line L45 (6, 39) -> (-1, 39)
  line L46 (-1, 39) -> (-1, 38.5)
  line L47 (-1, 38.5) -> (-3.5, 38.5)
  line L48 (-3.5, 38.5) -> (-3.5, 36.5)
  line L49 (-3.5, 36.5) -> (-5.5, 36.5)
  line L50 (-5.5, 36.5) -> (-5.5, 34)
  line L51 (-5.5, 34) -> (-6, 34)
  line L52 (-6, 34) -> (-6, 39)
  line L53 (-6, 39) -> (-1, 39)
  line L54 (-1, 39) -> (-1, 68)
  line L55 (-1, 68) -> (-0.5, 68)
  line L56 (-116.5, 3.5) -> (-116.5, 5.5)
  line L57 (-116.5, 5.5) -> (-114.5, 5.5)
  line L58 (-114.5, 5.5) -> (-114.5, 8)
  line L59 (-114.5, 8) -> (-114, 8)
  line L60 (-114, 8) -> (-114, 3)
  line L61 (-114, 3) -> (-119, 3)
  line L62 (-119, 3) -> (-119, 3.5)
  line L63 (-119, 3.5) -> (-116.5, 3.5)
  circle A0 centre (-9.9603, 7.5483) radius 1.25
  circle A1 centre (-111.4603, 7.5483) radius 1.25
  circle A2 centre (-9.9603, 64.0483) radius 1.25
  circle A3 centre (-111.4603, 64.0483) radius 1.25
  line L64 (8.5, 4.5) -> (8.5, 6.5)
  line L65 (8.5, 6.5) -> (10.5, 6.5)
  line L66 (10.5, 6.5) -> (10.5, 9)
  line L67 (10.5, 9) -> (11, 9)
  line L68 (11, 9) -> (11, 4)
  line L69 (11, 4) -> (6, 4)
  line L70 (6, 4) -> (6, 4.5)
  line L71 (6, 4.5) -> (8.5, 4.5)
  line L72 (-3.5, 6.5) -> (-3.5, 4.5)
  line L73 (-3.5, 4.5) -> (-1, 4.5)
  line L74 (-1, 4.5) -> (-1, 4)
  line L75 (-1, 4) -> (-6, 4)
  line L76 (-6, 4) -> (-6, 8.9372)
  line L77 (-6, 8.9372) -> (-5.5, 8.9372)
  line L78 (-5.5, 8.9372) -> (-5.5, 6.5)
  line L79 (-5.5, 6.5) -> (-3.5, 6.5)
  line L80 (-119.094, 68) -> (-130, 68)
  line L81 (-130, 68) -> (-130, 68.5)
  line L82 (-130, 68.5) -> (-119.094, 68.5)
  line L83 (-119.094, 68.5) -> (-119.094, 68)
  constraint horizontal L80
  constraint vertical L81
  constraint horizontal L82
  constraint vertical L83
  constraint coincident L19.end L20.start
  constraint coincident L17.end L18.start
extrude "Extrusion41" add sketch "Skizze41" along normal blind 10 separate body contours L18 L19 L20 L80 L81 L82 L83 makes body 4
sketch "Skizze42" plane through (0, 1, 0) normal (0, 1, 0) x (-1, 0, 0)
  line L0 (-0.5, 68) -> (-0.5, 39.5)
  line L1 (-0.5, 39.5) -> (16.5, 39.5)
  line L2 (16.5, 39.5) -> (16.5, 0.5)
  line L3 (16.5, 0.5) -> (-134.5, 0.5)
  line L4 (-134.5, 0.5) -> (-134.5, 3)
  line L5 (-134.5, 3) -> (-135, 3)
  line L6 (-135, 3) -> (-135, 0)
  line L7 (-135, 0) -> (17, 0)
  line L8 (17, 0) -> (17, 40)
  line L9 (17, 40) -> (0, 40)
  line L10 (0, 40) -> (0, 68.5)
  line L11 (0, 68.5) -> (-114.094, 68.5)
  line L12 (-114.094, 68.5) -> (-114.094, 63.5)
  line L13 (-114.094, 63.5) -> (-114.594, 63.5)
  line L14 (-114.594, 63.5) -> (-114.594, 66)
  line L15 (-114.594, 66) -> (-116.594, 66)
  line L16 (-116.594, 66) -> (-116.594, 68)
  line L17 (-116.594, 68) -> (-119.094, 68)
  line L18 (-119.094, 68) -> (-119.094, 68.5)
  line L19 (-119.094, 68.5) -> (-130, 68.5)
  line L20 (-130, 68.5) -> (-130, 68)
  line L21 (-130, 68) -> (-132.5, 68)
  line L22 (-132.5, 68) -> (-132.5, 66)
  line L23 (-132.5, 66) -> (-134.5, 66)
  line L24 (-134.5, 66) -> (-134.5, 63.5)
  line L25 (-134.5, 63.5) -> (-135, 63.5)
  line L26 (-135, 63.5) -> (-135, 8.5)
  line L27 (-135, 8.5) -> (-134.5, 8.5)
  line L28 (-134.5, 8.5) -> (-134.5, 5.5)
  line L29 (-134.5, 5.5) -> (-132.5, 5.5)
  line L30 (-132.5, 5.5) -> (-132.5, 3.5)
  line L31 (-132.5, 3.5) -> (-130, 3.5)
  line L32 (-130, 3.5) -> (-130, 3)
  line L33 (-130, 3) -> (-134, 3)
  line L34 (-134, 3) -> (-134, 1)
  line L35 (-134, 1) -> (16, 1)
  line L36 (16, 1) -> (16, 39)
  line L37 (16, 39) -> (11, 39)
  line L38 (11, 39) -> (11, 34)
  line L39 (11, 34) -> (10.5, 34)
  line L40 (10.5, 34) -> (10.5, 36.5)
  line L41 (10.5, 36.5) -> (8.5, 36.5)
  line L42 (8.5, 36.5) -> (8.5, 38.5)
  line L43 (8.5, 38.5) -> (6, 38.5)
  line L44 (6, 38.5) -> (6, 39)
  line L45 (6, 39) -> (-1, 39)
  line L46 (-1, 39) -> (-1, 38.5)
  line L47 (-1, 38.5) -> (-3.5, 38.5)
  line L48 (-3.5, 38.5) -> (-3.5, 36.5)
  line L49 (-3.5, 36.5) -> (-5.5, 36.5)
  line L50 (-5.5, 36.5) -> (-5.5, 34)
  line L51 (-5.5, 34) -> (-6, 34)
  line L52 (-6, 34) -> (-6, 39)
  line L53 (-6, 39) -> (-1, 39)
  line L54 (-1, 39) -> (-1, 68)
  line L55 (-1, 68) -> (-0.5, 68)
  line L56 (-116.5, 3.5) -> (-116.5, 5.5)
  line L57 (-116.5, 5.5) -> (-114.5, 5.5)
  line L58 (-114.5, 5.5) -> (-114.5, 8)
  line L59 (-114.5, 8) -> (-114, 8)
  line L60 (-114, 8) -> (-114, 3)
  line L61 (-114, 3) -> (-119, 3)
  line L62 (-119, 3) -> (-119, 3.5)
  line L63 (-119, 3.5) -> (-116.5, 3.5)
  circle A0 centre (-9.9603, 7.5483) radius 1.25
  circle A1 centre (-111.4603, 7.5483) radius 1.25
  circle A2 centre (-9.9603, 64.0483) radius 1.25
  circle A3 centre (-111.4603, 64.0483) radius 1.25
  line L64 (8.5, 4.5) -> (8.5, 6.5)
  line L65 (8.5, 6.5) -> (10.5, 6.5)
  line L66 (10.5, 6.5) -> (10.5, 9)
  line L67 (10.5, 9) -> (11, 9)
  line L68 (11, 9) -> (11, 4)
  line L69 (11, 4) -> (6, 4)
  line L70 (6, 4) -> (6, 4.5)
  line L71 (6, 4.5) -> (8.5, 4.5)
  line L72 (-3.5, 6.5) -> (-3.5, 4.5)
  line L73 (-3.5, 4.5) -> (-1, 4.5)
  line L74 (-1, 4.5) -> (-1, 4)
  line L75 (-1, 4) -> (-6, 4)
  line L76 (-6, 4) -> (-6, 8.9372)
  line L77 (-6, 8.9372) -> (-5.5, 8.9372)
  line L78 (-5.5, 8.9372) -> (-5.5, 6.5)
  line L79 (-5.5, 6.5) -> (-3.5, 6.5)
sketch "Skizze43" plane through (0, 4, 0) normal (0, 1, 0) x (-1, 0, 0)
  line L0 (-114.094, 63.5) -> (-114.094, 68.5)
  line L1 (-114.094, 68.5) -> (-119.094, 68.5)
  line L2 (-119.094, 68.5) -> (-119.094, 68)
  line L3 (-119.094, 68) -> (-114.594, 68)
  line L4 (-114.594, 68) -> (-114.594, 63.5)
  line L5 (-114.594, 63.5) -> (-114.094, 63.5)
  line L6 (-119.094, 68) -> (-114.094, 68)
  line L7 (-114.094, 68) -> (-114.094, 68.5)
  line L8 (-114.094, 68.5) -> (-119.094, 68.5)
  line L9 (-119.094, 68.5) -> (-119.094, 68)
  constraint horizontal L6
  constraint vertical L7
  constraint horizontal L8
  constraint vertical L9
  constraint coincident L0.end L1.start
  constraint coincident L2.end L3.start
extrude "Extrusion42" add sketch "Skizze43" along normal blind 7 contours L0 L1 L2 L3 L6 L7 L8 L9 bodies 4 1 3
sketch "Skizze44" plane through (0, 4, 0) normal (0, 1, 0) x (-1, 0, 0)
  line L0 (-114.094, 68) -> (-114.594, 68)
  line L1 (-114.594, 68) -> (-114.594, 63.5)
  line L2 (-114.594, 63.5) -> (-114.094, 63.5)
  line L3 (-114.094, 63.5) -> (-114.094, 67.5)
  line L4 (-114.094, 67.5) -> (-114.094, 68)
  line L5 (-114.094, 67.5) -> (-114.594, 67.5)
  line L6 (-114.594, 67.5) -> (-114.594, 68)
  line L7 (-114.594, 68) -> (-114.094, 68)
  line L8 (-114.094, 68) -> (-114.094, 67.5)
  constraint horizontal L5
  constraint vertical L6
  constraint horizontal L7
  constraint vertical L8
  constraint coincident L0.end L1.start
  constraint coincident L3.end L4.start
extrude "Extrusion43" add sketch "Skizze44" along normal blind 7 separate body contours L0 L1 L4 L5 L6 L7 L8 makes body 5
combine "Kombinieren1" operation add target body 4 tool bodies 5
sketch "Skizze45" plane through (0, 4, 0) normal (0, 1, 0) x (-1, 0, 0)
  line L0 (-135, 63.5) -> (-134.5, 63.5)
  line L1 (-134.5, 63.5) -> (-134.5, 68)
  line L2 (-134.5, 68) -> (-130, 68)
  line L3 (-130, 68) -> (-130, 68.5)
  line L4 (-130, 68.5) -> (-135, 68.5)
  line L5 (-135, 68.5) -> (-135, 63.5)
extrude "Extrusion44" add sketch "Skizze45" along normal blind 7 separate body makes body 6
sketch "Skizze46" plane through (0, 1, 0) normal (0, 1, 0) x (-1, 0, 0)
  line L0 (-135, 63.5) -> (-134.5, 63.5)
  line L1 (-134.5, 63.5) -> (-134.5, 8.5)
  line L2 (-134.5, 8.5) -> (-135, 8.5)
  line L3 (-135, 8.5) -> (-135, 63.5)
  constraint horizontal L0
  constraint vertical L1
  constraint horizontal L2
  constraint vertical L3
extrude "Extrusion45" add sketch "Skizze46" along normal blind 10 bodies 6 4
sketch "Skizze47" plane through (0, 4, 0) normal (0, 1, 0) x (-1, 0, 0)
  line L0 (-135, 8.5) -> (-135, 3)
  line L1 (-135, 3) -> (-134.5, 3)
  line L2 (-134.5, 3) -> (-134, 3)
  line L3 (-134, 3) -> (-130, 3)
  line L4 (-130, 3) -> (-130, 3.5)
  line L5 (-130, 3.5) -> (-134.5, 3.5)
  line L6 (-134.5, 3.5) -> (-134.5, 8.5)
  line L7 (-134.5, 8.5) -> (-135, 8.5)
  line L8 (-134.5, 3) -> (-135, 3)
  line L9 (-135, 3) -> (-135, 8.5)
  line L10 (-135, 8.5) -> (-134.5, 8.5)
  line L11 (-134.5, 8.5) -> (-134.5, 3)
  constraint horizontal L8
  constraint vertical L9
  constraint horizontal L10
  constraint vertical L11
  constraint coincident L0.start L7.end
  constraint coincident L1.end L2.start
extrude "Extrusion46" add sketch "Skizze47" along normal blind 7 separate body contours L0 L1 L6 L7 L8 L9 L10 L11 makes body 7
sketch "Skizze48" plane through (0, 4, 0) normal (0, 1, 0) x (-1, 0, 0)
  line L0 (-135, 8.5) -> (-135, 3)
  line L1 (-135, 3) -> (-134.5, 3)
  line L2 (-134.5, 3) -> (-134, 3)
  line L3 (-134, 3) -> (-130, 3)
  line L4 (-130, 3) -> (-130, 3.5)
  line L5 (-130, 3.5) -> (-134.5, 3.5)
  line L6 (-134.5, 3.5) -> (-134.5, 8.5)
  line L7 (-134.5, 8.5) -> (-135, 8.5)
sketch "Skizze49" plane through (0, 4, 0) normal (0, 1, 0) x (-1, 0, 0)
  line L0 (-134, 3) -> (-134.5, 3)
  line L1 (-134.5, 3) -> (-134.5, 3.5)
  line L2 (-134.5, 3.5) -> (-134, 3.5)
  line L3 (-134, 3.5) -> (-134, 3)
  constraint horizontal L0
  constraint vertical L1
  constraint horizontal L2
  constraint vertical L3
extrude "Extrusion47" add sketch "Skizze49" along normal blind 7 bodies 7 6
